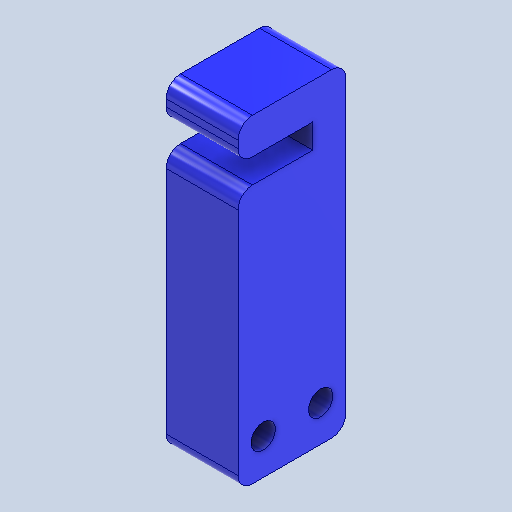
# Autodesk Inventor part: base_weel-v2-3DP-C-F-3
Saved by Autodesk Inventor 2025.2 (Build 292293000, 293)
## iProperties
Created: 2025-01-15
Part Number: base_weel-v2-3DP-C-F-3
Material: ABS プラスチック
Document SubType Name: Modeling
Designer: haruy
Density: 1.06 g/cm^3
Appearance: 青 - 壁塗料 - 光沢
Author: haruy
Autodesk Inventor part; units mm, degrees
ref_plane "YZ Plane" through (0, 0, 0) normal (1, 0, 0) x (0, 1, 0)
ref_plane "XZ Plane" through (0, 0, 0) normal (0, 1, 0) x (-1, 0, 0)
ref_plane "XY Plane" through (0, 0, 0) normal (0, 0, 1) x (1, 0, 0)
sketch "スケッチ1" plane through (0, 0, 0) normal (1, 0, 0) x (0, 1, 0)
  line L0 (0, 0) -> (3.4, 0)
  line L1 (3.4, 0) -> (3.4, -83.525)
  line L2 (3.4, -83.525) -> (0, -83.525)
  line L3 (0, -83.525) -> (0, 0)
  line L4 (-26, 0) -> (-36, 0)
  line L5 (-36, 0) -> (-36, -134.3533)
  line L6 (-36, -134.3533) -> (-26, -134.3533)
  line L7 (-26, -134.3533) -> (-26, 0)
  line L8 (3.4, -83.525) -> (8.4, -83.525)
  line L9 (8.4, -83.525) -> (8.4, -73.125)
  line L10 (8.4, -73.125) -> (3.4, -73.125)
  line L11 (3.4, -73.125) -> (3.4, -83.525)
  line L12 (0, -73.125) -> (-36, -73.125)
  line L13 (-36, -73.125) -> (-36, -88.125)
  line L14 (-36, -88.125) -> (0, -88.125)
  line L15 (0, -88.125) -> (0, -73.125)
  line L16 (8.4, -83.525) -> (0, -83.525)
  line L17 (0, -83.525) -> (0, -88.125)
  line L18 (0, -88.125) -> (8.4, -88.125)
  line L19 (8.4, -88.125) -> (8.4, -83.525)
  circle A0 centre (-31, -76.625) radius 1.7
  circle A1 centre (-31, -84.625) radius 1.7
  point P0 (4.2, -88.125)
  point P1 (5.9, -83.525)
  point P2 (-36, -80.625)
  point P3 (3.4, -73.125)
  point P4 (-36, -73.125)
  dimension "d0" = 3.4
  dimension "d1" = 10
  dimension "d2" = 26
  dimension "d3" = 5
  dimension "d4" = 10.4
  dimension "d5" = 4.6
  dimension "d6" = 3.4
  dimension "d7" = 3.4
  dimension "d8" = 5
  dimension "d9" = 5
  dimension "d10" = 8
  dimension "d11" = 3.5
  dimension "d14" = 0
  constraints: 40 end point, 10 parallel, 5 horizontal, 5 perpendicular, 3 midpoint, 3 point on line, 2 centre point
  measures "d0" distance of L1.end L2.end
  measures "d1" distance of L6.end L5.end
  measures "d2" distance between parallel lines of L7 L3
  measures "d3" distance of L10.end L9.end
  measures "d4" distance of L8.end L9.end
  measures "d5" vertical distance of point (4.2, -88.125) point (5.9, -83.525)
  measures "d6" diameter of A0
  measures "d7" diameter of A1
  measures "d8" distance from line of A0.centre L13
  measures "d9" horizontal distance of A1.centre point (-36, -80.625)
  measures "d10" distance of A1.centre A0.centre
  measures "d11" distance from line of A0.centre L12
  measures "d14" distance between parallel lines of L10 L12
extrude "押し出し1" add sketch "スケッチ1" against normal blind 10 contours L3 L15 L14 L7 L12 | L10 L9 L8 L1 | L2 L8 L19 L18 L15 | L7 L14 L5 L12
fillet "フィレット1" radius 2 6 edges at (-5, -36, -88.125) (-5, -36, -73.125) (-5, 0, -73.125) (-5, 3.4, -73.125) (-5, 8.4, -73.125) (-5, 8.4, -88.125)
equation "\"d9\" = d8"
